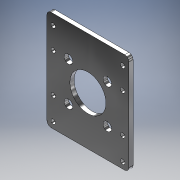
# Autodesk Inventor part: ハンド_シリンダ固定板
Saved by Autodesk Inventor 2019.4 (Build 234330000, 330)
## iProperties
Created: 2021-12-05
Part Number: ハンド_シリンダ固定板
Material: アルミニウム 6061
Document SubType Name: Modeling
Designer: 堀川皓史
Density: 2.7 g/cm^3
Appearance: アルミニウム - フラット
Author: 堀川皓史
Autodesk Inventor part; units mm, degrees
ref_plane "YZ Plane" through (0, 0, 0) normal (1, 0, 0) x (0, 1, 0)
ref_plane "XZ Plane" through (0, 0, 0) normal (0, 1, 0) x (-1, 0, 0)
ref_plane "XY Plane" through (0, 0, 0) normal (0, 0, 1) x (1, 0, 0)
sketch "スケッチ1" plane through (0, 0, 0) normal (0, 0, 1) x (1, 0, 0)
  circle A0 centre (0, 0) radius 13
  circle A1 centre (-14, 14) radius 3.1
  circle A2 centre (14, 14) radius 3.1
  circle A3 centre (-14, -14) radius 3.1
  circle A4 centre (14, -14) radius 3.1
  line L0 (20, 20) -> (-20, 20) construction
  line L1 (-20, 20) -> (-20, -20) construction
  line L2 (-20, -20) -> (20, -20) construction
  line L3 (20, -20) -> (20, 20) construction
  line L4 (20, 20) -> (-20, -20) construction
  line L5 (-20, 20) -> (20, -20) construction
  circle A5 centre (-25, 14) radius 1.6
  circle A6 centre (-25, -14) radius 1.6
  circle A7 centre (25, 14) radius 1.6
  circle A8 centre (25, -14) radius 1.6
  line L6 (-47.387, 37) -> (51.5127, 37) construction
  line L7 (51.5127, 37) -> (51.5127, 22) construction
  line L8 (51.5127, 22) -> (-47.387, 22) construction
  line L9 (-47.387, 22) -> (-47.387, 37) construction
  circle A9 centre (-25, 29.5) radius 1.6
  circle A10 centre (25, 29.5) radius 1.6
  circle A11 centre (-25, -30.5) radius 1.6
  circle A12 centre (25, -30.5) radius 1.6
  line L10 (-36.8919, -26) -> (36.9631, -26) construction
  line L11 (36.9631, -26) -> (36.9631, -35) construction
  line L12 (36.9631, -35) -> (-36.8919, -35) construction
  line L13 (-36.8919, -35) -> (-36.8919, -26) construction
  line L14 (-29.5, 37) -> (-29.5, -35)
  line L15 (-29.5, 37) -> (29.5, 37)
  line L16 (29.5, 37) -> (29.5, -35)
  line L17 (-29.5, -35) -> (29.5, -35)
  dimension "d0" = 26
  dimension "d1" = 6.2
  dimension "d2" = 6.2
  dimension "d3" = 6.2
  dimension "d4" = 6.2
  dimension "d5" = 28
  dimension "d6" = 28
  dimension "d7" = 14
  dimension "d8" = 14
  dimension "d9" = 40
  dimension "d10" = 40
  dimension "d11" = 3.2
  dimension "d12" = 3.2
  dimension "d13" = 3.2
  dimension "d14" = 3.2
  dimension "d15" = 15
  dimension "d16" = 2
  dimension "d17" = 5
  dimension "d18" = 5
  dimension "d19" = 3.2
  dimension "d20" = 3.2
  dimension "d21" = 7.5
  dimension "d22" = 3.2
  dimension "d23" = 3.2
  dimension "d26" = 9
  dimension "d27" = 4.5
  dimension "d28" = 63
  dimension "d29" = 4.5
  dimension "d30" = 4.5
  constraints: 36 end point, 13 centre point, 8 horizontal alignment, 8 vertical alignment, 6 parallel, 6 perpendicular, 4 point on line, 3 horizontal, 2 midpoint, 1 coincident
  measures "d0" diameter of A0
  measures "d1" diameter of A1
  measures "d2" diameter of A2
  measures "d3" diameter of A3
  measures "d4" diameter of A4
  measures "d5" distance of A3.centre A1.centre
  measures "d6" distance of A1.centre A2.centre
  measures "d7" horizontal distance of point (0, 0) A1.centre
  measures "d8" horizontal distance of point (0, 0) A1.centre
  measures "d9" distance of L2.end L1.end
  measures "d10" distance of L1.end L0.end
  measures "d11" diameter of A5
  measures "d12" diameter of A6
  measures "d13" diameter of A7
  measures "d14" diameter of A8
  measures "d15" distance between parallel lines of L8 L6
  measures "d16" distance between parallel lines of L0 L8
  measures "d17" distance from line of L1 A5.centre
  measures "d18" distance from line of L3 A7.centre
  measures "d19" diameter of A9
  measures "d20" diameter of A10
  measures "d21" distance from line of L6 A9.centre
  measures "d22" diameter of A11
  measures "d23" diameter of A12
  measures "d26" distance of L12.end L10.start
  measures "d27" distance from line of A11.centre L10
  measures "d28" distance between parallel lines of L10 L6
  measures "d29" distance from line of L16 A7.centre
  measures "d30" distance from line of A5.centre L14
extrude "押し出し1" add sketch "スケッチ1" along normal blind 3
fillet "フィレット1" radius 3 4 edges at (-29.5, 37, 1.5) (29.5, 37, 1.5) (29.5, -35, 1.5) (-29.5, -35, 1.5)
equation "\"d7\" = 0.5 * d5"
equation "\"d8\" = 0.5 * d6"
